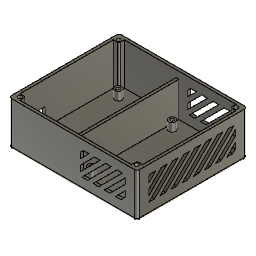
case (Autodesk Fusion 360 design; units mm, degrees)
Autodesk Fusion 360 part; units mm, degrees
sketch "Skizze1" plane through (0, 0, 0) normal (0, 0, 1) x (1, 0, 0)
  line L0 (0, 0) -> (88, 0)
  line L1 (88, 0) -> (88, 75)
  line L2 (88, 75) -> (0, 75)
  line L3 (0, 75) -> (0, 0)
  line L4 (0, 5) -> (88, 5) construction
  line L5 (83, 0) -> (83, 75) construction
  line L6 (48, 0) -> (48, 75) construction
  line L7 (43, 0) -> (43, 75)
  line L8 (41, 0) -> (41, 75)
  line L9 (88, 70) -> (0, 70) construction
  line L10 (8, 75) -> (8, 0) construction
  line L11 (88, 66.5) -> (0, 66.5) construction
  circle A0 centre (8, 66.5) radius 1.25
  line L12 (28.5, 75) -> (28.5, 0) construction
  circle A1 centre (28.5, 66.5) radius 1.25
  circle A2 centre (28.5, 66.5) radius 2.5
  circle A3 centre (8, 66.5) radius 2.5
  line L13 (32, 75) -> (32, 0) construction
  line L14 (0, 8.5) -> (88, 8.5) construction
  circle A4 centre (8, 8.5) radius 1.25
  circle A5 centre (28.5, 8.5) radius 1.25
  circle A6 centre (8, 8.5) radius 2.5
  circle A7 centre (28.5, 8.5) radius 2.5
  line L15 (2, 75) -> (2, 0) construction
  circle A8 centre (28.5, 66.5) radius 1.25
  circle A9 centre (28.5, 66.5) radius 2.5
  circle A10 centre (28.5, 66.5) radius 2.5
  circle A11 centre (28.5, 66.5) radius 1.25
  circle A12 centre (28.5, 66.5) radius 1.25
  circle A13 centre (28.5, 66.5) radius 2.5
  circle A14 centre (28.5, 66.5) radius 2.5
  circle A15 centre (46.7, 66.5) radius 2.5
  circle A16 centre (46.7, 66.5) radius 1.25
  circle A17 centre (46.7, 8.5) radius 2.5
  circle A18 centre (46.7, 8.5) radius 1.25
  circle A19 centre (84.3, 8.5) radius 1.25
  circle A20 centre (84.3, 8.5) radius 2.5
  circle A21 centre (84.3, 66.5) radius 2.5
  circle A22 centre (84.3, 66.5) radius 1.25
  line L16 (88, 71) -> (0, 71)
  line L17 (4, 75) -> (4, 0)
  line L18 (0, 4) -> (88, 4)
  line L19 (84, 0) -> (84, 75)
  line L20 (0, 71) -> (4, 75) construction
  line L21 (4, 71) -> (0, 75) construction
  circle A23 centre (2, 73) radius 1.5
  line L22 (4, 4) -> (0, 0) construction
  line L23 (0, 4) -> (4, 0) construction
  circle A24 centre (2, 2) radius 1.5
  line L24 (88, 4) -> (84, 0) construction
  line L25 (84, 4) -> (88, 0) construction
  circle A25 centre (86, 2) radius 1.5
  line L26 (84, 71) -> (88, 75) construction
  line L27 (84, 75) -> (88, 71) construction
  circle A26 centre (86, 73) radius 1.5
  dimension "d1" = 88
  dimension "d2" = 75
  dimension "d4" = -5
  dimension "d6" = -5
  dimension "d7" = -40
  dimension "d15" = -5
  dimension "d18" = 2.5
  dimension "d20" = 2.5
  dimension "d21" = 5
  dimension "d22" = 5
  dimension "d25" = 2.5
  dimension "d26" = 2.5
  dimension "d27" = 5
  dimension "d28" = 5
  dimension "d29" = -2
  dimension "d30" = 2.5
  dimension "d31" = 5
  dimension "d32" = 2.5
  dimension "d33" = 5
  dimension "d34" = 2.5
  dimension "d35" = 5
  dimension "d36" = 5
  dimension "d37" = 2.5
  dimension "d38" = 5
  dimension "d39" = 2.5
  dimension "d40" = 5
  dimension "d41" = 2.5
  dimension "d42" = 5
  dimension "d43" = 5
  dimension "d44" = 2.5
  dimension "d92" = -4
  dimension "d93" = -4
  dimension "d94" = -4
  dimension "d95" = -4
  dimension "d96" = 3
  dimension "d97" = 3
  dimension "d98" = 3
  dimension "d99" = 3
  constraint horizontal L0
  constraint vertical L1
  constraint horizontal L2
  constraint vertical L3
  constraint coincident L0.start L3.end
  constraint coincident L11 A0.centre
  constraint coincident L10 A0.centre
  constraint coincident L12 A1.centre
  constraint coincident L11 A1.centre
  constraint concentric A1 A2
  constraint concentric A0 A3
  constraint coincident L10 A4.centre
  constraint coincident L14 A4.centre
  constraint coincident L14 A5.centre
  constraint coincident L12 A5.centre
  constraint concentric A4 A6
  constraint concentric A5 A7
  constraint concentric A8 A9
  constraint concentric A10 A11
  constraint concentric A17 A18
  constraint concentric A19 A20
  constraint coincident L16 L21.start
  constraint coincident L17 L21.start
  constraint perpendicular L20 L21
  constraint midpoint L20 A23.centre
  constraint coincident L18 L22.start
  constraint coincident L17 L22.start
  constraint perpendicular L22 L23
  constraint midpoint L23 A24.centre
  constraint coincident L18 L25.start
  constraint coincident L19 L25.start
  constraint perpendicular L24 L25
  constraint midpoint L25 A25.centre
  constraint coincident L16 L26.start
  constraint coincident L19 L26.start
  constraint perpendicular L26 L27
  constraint midpoint L26 A26.centre
  measures "d1" distance of L0.start L0.end
  measures "d2" distance of L0.start L2.end
  measures "d18" diameter of A0
  measures "d20" diameter of A1
  measures "d21" diameter of A2
  measures "d22" diameter of A3
  measures "d25" diameter of A4
  measures "d26" diameter of A5
  measures "d27" diameter of A6
  measures "d28" diameter of A7
  measures "d30" diameter of A8
  measures "d31" diameter of A9
  measures "d32" diameter of A11
  measures "d33" diameter of A10
  measures "d34" diameter of A12
  measures "d35" diameter of A13
  measures "d36" diameter of A14
  measures "d37" diameter of A16
  measures "d38" diameter of A15
  measures "d39" diameter of A18
  measures "d40" diameter of A17
  measures "d41" diameter of A19
  measures "d42" diameter of A20
  measures "d43" diameter of A21
  measures "d44" diameter of A22
  measures "d96" diameter of A23
  measures "d97" diameter of A24
  measures "d98" diameter of A25
  measures "d99" diameter of A26
extrude "Extrusion1" add sketch "Skizze1" along normal blind 30 contours L0 L3 L17 L18 | L0 L8 L17 L18 | L3 L16 L17 L18 | L0 L7 L8 L18 | L8 L16 L17 L18 | L2 L3 L16 L17 | L0 L7 L18 L19 | L7 L8 L16 L18 | L2 L8 L16 L17 | L0 L1 L18 L19 | L7 A20 A21 L16 L18 L19 | L2 L7 L8 L16 | L1 A20 A21 L16 L18 L19 | L2 L7 L16 L19 | A19 A20 L19 | A19 A20 L19 | L1 L2 L16 L19 | A19 L19 | A19 L19 | A21 A22 L19 | A21 A22 L19 | A22 L19 | A22 L19 | A0 | A1 A8 A11 A12 | A2 A9 A10 A13 A14 | A3 | A4 | A5 | A6 | A7 | A15 | A16 | A17 | A18 | A23 | A24 | A25 | A26 makes body 1
shell "Schale1" thickness 2 outward yes removed faces 0 bodies 1
ref_plane "Arbeitsebene1" through (44, 37.5, 30) normal (0, 0, 1) x (1, 0, 0)
split "Teilen1" by plane through (44, 37.5, 30) normal (0, 0, 1) bodies 1 makes body 2 at (28.6667, 24.3333, 32)
extrude "Extrusion2" add sketch "Skizze1" along normal blind 6 contours A19 A20 L19 | A19 A20 L19 | A21 A22 L19 | A21 A22 L19 | A2 A9 A10 A13 A14 | A3 | A6 | A7 | A15 | A17 bodies 1
extrude "Extrusion3" add sketch "Skizze1" along normal blind 25 contours L0 L7 L8 L18 | L7 L8 L16 L18 | L2 L7 L8 L16 bodies 1
fillet "Abrundung1" radius 2 4 edges at (90, -2, 14) (-2, -2, 14) (-2, 77, 14) (90, 77, 14) on bodies 1
fillet "Abrundung2" radius 2 8 edges at (-2, 37.5, -2) (-1.4142, -1.4142, -2) (44, -2, -2) (89.4142, -1.4142, -2) (90, 37.5, -2) (89.4142, 76.4142, -2) (44, 77, -2) (-1.4142, 76.4142, -2) on bodies 1
sketch "Skizze2" plane through (-2, 0, 0) normal (-1, 0, 0) x (0, -1, 0)
  line L0 (-75, 0) -> (0, 0)
  line L1 (0, 0) -> (0, 30)
  line L2 (0, 30) -> (-75, 30)
  line L3 (-75, 30) -> (-75, 0)
  line L4 (-75, 13) -> (0, 13)
  line L5 (-75, 4) -> (0, 4)
  line L6 (-70, 30) -> (-70, 0) construction
  line L7 (-16, 30) -> (-16, 0) construction
  line L8 (-22, 30) -> (-22, 0)
  line L9 (-10, 30) -> (-10, 0)
  dimension "d61" = -13
  dimension "d62" = -4
  dimension "d63" = -5
  dimension "d64" = -59
  dimension "d65" = -53
  dimension "d66" = -65
extrude "Extrusion4" cut sketch "Skizze2" against normal blind 5 contours L4 L5 L8 L9 bodies 1
sketch "Skizze3" plane through (90, 0, 0) normal (1, 0, 0) x (0, 1, 0)
  line L0 (0, 0) -> (75, 0)
  line L1 (75, 0) -> (75, 30)
  line L2 (75, 30) -> (0, 30)
  line L3 (0, 30) -> (0, 0)
  line L4 (0, 0) -> (28.8843, 28.8843)
  line L5 (0, 0) -> (40.8486, 0) construction
  line L6 (4, 0) -> (32.8843, 28.8843)
  line L7 (8, 0) -> (36.8843, 28.8843)
  line L8 (12, 0) -> (40.8843, 28.8843)
  line L9 (28, 0) -> (56.8843, 28.8843)
  line L10 (24, 0) -> (52.8843, 28.8843)
  line L11 (20, 0) -> (48.8843, 28.8843)
  line L12 (16, 0) -> (44.8843, 28.8843)
  line L13 (60, 0) -> (88.8843, 28.8843)
  line L14 (56, 0) -> (84.8843, 28.8843)
  line L15 (52, 0) -> (80.8843, 28.8843)
  line L16 (48, 0) -> (76.8843, 28.8843)
  line L17 (44, 0) -> (72.8843, 28.8843)
  line L18 (40, 0) -> (68.8843, 28.8843)
  line L19 (36, 0) -> (64.8843, 28.8843)
  line L20 (32, 0) -> (60.8843, 28.8843)
  line L21 (-20, 0) -> (8.8843, 28.8843)
  line L22 (-16, 0) -> (12.8843, 28.8843)
  line L23 (-12, 0) -> (16.8843, 28.8843)
  line L24 (-8, 0) -> (20.8843, 28.8843)
  line L25 (-4, 0) -> (24.8843, 28.8843)
  line L26 (64, 0) -> (92.8843, 28.8843)
  line L27 (68.5, 23.5) -> (6.5, 23.5)
  line L28 (6.5, 23.5) -> (6.5, 6.5)
  line L29 (6.5, 6.5) -> (68.5, 6.5)
  line L30 (68.5, 6.5) -> (68.5, 23.5)
  point P0 (10, 20)
  dimension "d79" = -6.5
  constraint horizontal L5
  constraint coincident L0.start L3.end
extrude "Extrusion5" cut sketch "Skizze3" against normal blind 2 contours L4 L6 L27 L29 | L24 L25 L27 L28 | L7 L8 L27 L29 | L22 L23 L27 L28 | L11 L12 L27 L29 | L9 L10 L27 L29 | L19 L20 L27 L29 | L15 L16 L29 L30 | L17 L18 L27 L29 | L13 L14 L29 L30 bodies 1
sketch "Skizze4" plane through (0, -2, 0) normal (0, -1, 0) x (1, 0, 0)
  line L0 (0, 0) -> (88, 0)
  line L1 (88, 0) -> (88, 30)
  line L2 (88, 30) -> (0, 30)
  line L3 (0, 30) -> (0, 0)
  line L4 (0, 0) -> (42.4264, 0) construction
  line L5 (16, 0) -> (46, 30)
  line L6 (20, 0) -> (50, 30)
  line L7 (24, 0) -> (54, 30)
  line L8 (28, 0) -> (58, 30)
  line L9 (32, 0) -> (62, 30)
  line L10 (36, 0) -> (66, 30)
  line L11 (40, 0) -> (70, 30)
  line L12 (44, 0) -> (74, 30)
  line L13 (48, 0) -> (78, 30)
  line L14 (52, 0) -> (82, 30)
  line L15 (56, 0) -> (86, 30)
  line L16 (60, 0) -> (90, 30)
  line L17 (84, 0) -> (114, 30)
  line L18 (80, 0) -> (110, 30)
  line L19 (76, 0) -> (106, 30)
  line L20 (72, 0) -> (102, 30)
  line L21 (68, 0) -> (98, 30)
  line L22 (64, 0) -> (94, 30)
  line L23 (43, 30) -> (43, 0)
  line L24 (43, 30) -> (88, 30)
  line L25 (88, 30) -> (88, 0)
  line L26 (88, 0) -> (43, 0)
  line L27 (43, 0) -> (43, 30)
  line L28 (81.5, 23.5) -> (81.5, 6.5)
  line L29 (81.5, 6.5) -> (49.5, 6.5)
  line L30 (49.5, 6.5) -> (49.5, 23.5)
  line L31 (49.5, 23.5) -> (81.5, 23.5)
  dimension "d85" = 6.5
  constraint horizontal L4
  constraint coincident L0.start L3.end
  constraint horizontal L24
  constraint vertical L25
  constraint horizontal L26
  constraint vertical L27
  constraint coincident L0.end L1.start
extrude "Extrusion6" cut sketch "Skizze4" against normal blind 95 contours L8 L9 L30 L31 | L10 L11 L30 L31 | L12 L13 L29 L31 | L14 L15 L29 L31 | L16 L22 L28 L29 | L20 L21 L28 L29 bodies 1
fillet "Abrundung3" radius 2 4 edges at (-2, -2, 31) (90, -2, 31) (90, 77, 31) (-2, 77, 31) on bodies 2
fillet "Abrundung4" radius 2 8 edges at (-1.4142, 76.4142, 32) (-2, 37.5, 32) (-1.4142, -1.4142, 32) (44, -2, 32) (89.4142, -1.4142, 32) (90, 37.5, 32) (89.4142, 76.4142, 32) (44, 77, 32) on bodies 2
extrude "Extrusion7" add sketch "Skizze1" along normal blind 30 contours L0 L3 L17 L18 | L2 L3 L16 L17 | L0 L1 L18 L19 | L1 L2 L16 L19 bodies 1
fillet "Abrundung5" radius 1 4 edges at (4, 71, 15) (84, 71, 15) (84, 4, 15) (4, 4, 15) on bodies 1
hidden bodies 2
